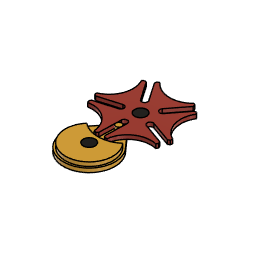
geneva_wheel (Autodesk Fusion 360 design; units mm, degrees)
part number: 2025-07-03-15-58-40-120
part number: 2025-07-03-15-58-53-115
part number: 2025-07-03-16-05-47-855
part number: 2025-07-03-16-28-11-939
Autodesk Fusion 360 part; units mm, degrees
note: some values were not read from the file. Set by a fixed rule: which sketch regions a step uses.
sketch "Sketch1" plane through (0, 0, 0) normal (0, 0, 1) x (1, 0, 0) in component "follower"
  line L0 (0, 0) -> (29.3893, -40.4508) construction
  line L1 (0, 0) -> (50, 0) construction
  line L2 (0, 0) -> (-29.3893, -40.4508) construction
  line L3 (0, 0) -> (50, 0) construction
  circle A0 centre (0, -65) radius 38.206 construction
  line L4 (8.7219, -18.3845) -> (26.3554, -42.655)
  line L5 (32.4231, -38.2467) -> (14.7895, -13.9761)
  arc A1 (14.7895, -13.9761) -> (8.7219, -18.3845) centre (11.7557, -16.1803) ccw
  line L6 (11.7557, -16.1803) -> (29.3893, -40.4508) construction
  line L7 (46.394, 19.0173) -> (17.8623, 9.7468)
  arc A2 (17.8623, 9.7468) -> (20.1799, 2.6139) centre (19.0211, 6.1803) ccw
  line L8 (20.1799, 2.6139) -> (48.7116, 11.8844)
  line L9 (-3.75, 50) -> (-3.75, 20)
  arc A3 (-3.75, 20) -> (3.75, 20) centre (0, 20) ccw
  line L10 (3.75, 20) -> (3.75, 50)
  line L11 (-48.7116, 11.8844) -> (-20.1799, 2.6139)
  arc A4 (-20.1799, 2.6139) -> (-17.8623, 9.7468) centre (-19.0211, 6.1803) ccw
  line L12 (-17.8623, 9.7468) -> (-46.394, 19.0173)
  line L13 (-26.3554, -42.655) -> (-8.7219, -18.3845)
  arc A5 (-8.7219, -18.3845) -> (-14.7895, -13.9761) centre (-11.7557, -16.1803) ccw
  line L14 (-14.7895, -13.9761) -> (-32.4231, -38.2467)
  circle A6 centre (0, 0) radius 7.5
  arc A7 (-29.3893, -40.4508) -> (-29.3183, -40.5023) centre (0, 0) ccw
  arc A8 (-26.2727, -42.5411) -> (-22.1872, -44.8077) centre (0, 0) ccw
  arc A9 (22.1872, -44.8077) -> (26.2727, -42.5411) centre (0, 0) ccw
  arc A10 (22.1872, -44.8077) -> (-22.1872, -44.8077) centre (0, -65) ccw
  arc A11 (49.4709, 7.2549) -> (35.7584, -34.9476) centre (61.8187, -20.0861) ccw
  arc A12 (8.3875, 49.2915) -> (44.2871, 23.2089) centre (38.206, 52.5861) ccw
  arc A13 (-44.2871, 23.2089) -> (-8.3875, 49.2915) centre (-38.206, 52.5861) ccw
  arc A14 (-35.7584, -34.9476) -> (-49.4709, 7.2549) centre (-61.8187, -20.0861) ccw
  arc A15 (-48.5777, 11.8409) -> (-49.4709, 7.2549) centre (0, 0) ccw
  arc A16 (-35.7584, -34.9476) -> (-32.3403, -38.1327) centre (0, 0) ccw
  arc A17 (-3.75, 49.8592) -> (-8.3875, 49.2915) centre (0, 0) ccw
  arc A18 (-44.2871, 23.2089) -> (-46.2601, 18.9738) centre (0, 0) ccw
  arc A19 (46.2601, 18.9738) -> (44.2871, 23.2089) centre (0, 0) ccw
  arc A20 (8.3875, 49.2915) -> (3.75, 49.8592) centre (0, 0) ccw
  arc A21 (32.3403, -38.1327) -> (35.7584, -34.9476) centre (0, 0) ccw
  arc A22 (50, 0) -> (48.5777, 11.8409) centre (0, 0) ccw
  dimension "d13" = 360
  constraint coincident L0.start L1.start
  constraint horizontal L1
  constraint horizontal L3
  constraint tangent L0 A0
  constraint tangent L2 A0
  constraint concentric A0 A10
  constraint parallel L4 L5
  constraint tangent L5 A1
  constraint tangent L4 A1
  constraint coincident L0.end L6.end
  constraint parallel L0 L6
  constraint concentric A6 A15
  constraint coincident L12 A18.end
  constraint coincident L11 A15.start
  constraint coincident L8 A22.end
  constraint coincident L7 A19.start
  constraint concentric A15 A19
  constraint coincident L10 A20.end
  constraint coincident L9 A17.start
  constraint concentric A17 A19
  constraint coincident L14 A16.end
  constraint concentric A7 A15
  constraint coincident A0 A7.end
  constraint coincident L13 A8.start
  constraint concentric A7 A8
  constraint coincident L4 A9.end
  constraint concentric A8 A21
  constraint coincident L5 A21.start
  constraint concentric A8 A9
  constraint concentric A15 A16
  constraint concentric A17 A18
  constraint concentric A19 A20
  constraint concentric A21 A22
  measures "d23" distance of L7.start
extrude "Extrude1" add sketch "Sketch1" along normal blind 5 makes body 1 in component "follower"
chamfer "Chamfer1" distance 2 angle 45 10 edges at (3.75, 49.8592, 2.5) (-3.75, 49.8592, 2.5) (46.2601, 18.9738, 2.5) (48.5777, 11.8409, 2.5) (26.2727, -42.5411, 2.5) (32.3403, -38.1327, 2.5) (-26.2727, -42.5411, 2.5) (-32.3403, -38.1327, 2.5) (-48.5777, 11.8409, 2.5) (-46.2601, 18.9738, 2.5) on bodies 1 in component "follower"
sketch "Sketch1 (2)" plane through (0, 0, 0) normal (0, 0, 1) x (1, 0, 0) in component "cam"
sketch "Sketch2" plane through (0, 0, 0) normal (0, 0, 1) x (1, 0, 0) in component "cam"
  circle A0 centre (0, -65) radius 38.206
  circle A1 centre (0, -65) radius 30
  circle A2 centre (0, -65) radius 32.5
  circle A3 centre (0, -65) radius 7.5
  circle A4 centre (-0.1016, -26.7941) radius 3.75
  line L0 (-24.6979, -43.875) -> (-3.7997, -19.4423)
  line L1 (3.7997, -19.4423) -> (24.6979, -43.875)
  arc A5 (3.7997, -19.4423) -> (-3.7997, -19.4423) centre (0, -22.6923) ccw
  arc A6 (-22.3607, -45) -> (22.3607, -45) centre (0, -18.0742) ccw
  point P0 (0, -15)
  dimension "d17" = 60
  dimension "d18" = 65
  dimension "d19" = 15
  dimension "d20" = 7.5
  dimension "d21" = 15
  dimension "d22" = 5
  dimension "d23" = 20
  dimension "d24" = 35
  constraint concentric A0 A1
  constraint concentric A0 A2
  constraint concentric A2 A3
  constraint coincident A0 A4.centre
  constraint coincident A2 L0.start
  constraint coincident A2 L1.end
  constraint tangent A2 L0
  constraint tangent A2 L1
  constraint vertical origin P0
  constraint coincident P0 L0
  constraint coincident P0 L1
  constraint tangent L0 A5
  constraint tangent L1 A5
  constraint coincident A1 A6.end
  constraint coincident A1 A6.start
  constraint horizontal A6.start A6.end
  measures "d17" diameter of A1
  measures "d18" diameter of A2
  measures "d19" diameter of A3
  measures "d20" diameter of A4
  measures "d21" distance of origin P0
  measures "d22" radius of A5
  measures "d23" vertical distance of A0.centre A6.start
  measures "d24" radius of A6
extrude "Extrude1'" add sketch "Sketch2" against normal blind 5 separate body contours A0 A2 A4 L0 L1 | A0 A4 L0 L1 A5 | A0 A4 | A0 A4 | A2 | A1 A6 | A1 A6 makes body 2 in component "cam"
extrude "Extrude2" add sketch "Sketch2" along normal blind 5 contours A0 A4 | A0 A4 | A1 A6 picked at (-16.7037, -56.5009) bodies 2 in component "cam"
cylinder "CylinderPrimitive1" add diameter 15 height -20 placed x (1, 0, 0) y (0, 1, 0) z (0, 0, 1) at (0, 0, 5) separate body makes body 3 in component "Component"
component "cam" placed x (0.999996, -0.002659, 0) y (0.002659, 0.999996, 0) z (0, 0, 1) at (0.1729, -0.0002, 0)
component "follower" placed x (0.809017, 0.587785, 0) y (-0.587785, 0.809017, 0) z (0, 0, 1) at (0, 0, 0)
component "Component" placed x (1, 0, 0) y (0, 1, 0) z (0, 0, 1) at (0, 0, 0)
component "Component" placed x (1, 0, 0) y (0, 1, 0) z (0, 0, 1) at (0, -65, 0)
